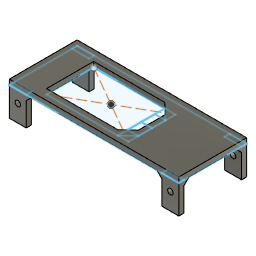
Power Rear Panel (Autodesk Fusion 360 design; units mm, degrees)
Autodesk Fusion 360 part; units mm, degrees
sketch "Sketch1" plane through (0, 0, 0) normal (0, 0, 1) x (1, 0, 0)
  line L0 (17.85, 0) -> (24.15, 0)
  line L1 (24.15, -8) -> (17.85, -13.9)
  line L2 (17.85, 8) -> (17.85, 0)
  line L3 (17.85, -13.9) -> (17.85, 13.9)
  line L4 (17.85, -8) -> (17.85, 0)
  line L5 (17.85, 0) -> (24.15, 0)
  line L6 (17.85, 13.9) -> (-24.15, 13.9)
  line L7 (24.15, 0) -> (24.15, -8)
  line L8 (-24.15, 13.9) -> (24.15, -13.9) construction
  line L9 (24.15, 8) -> (23.8007, 8)
  line L10 (24.15, -8) -> (17.85, -8)
  line L11 (24.15, 8) -> (17.85, 8)
  line L12 (24.15, 0) -> (24.15, 8)
  line L13 (17.85, 13.9) -> (24.15, 8)
  line L14 (-24.15, 13.9) -> (24.15, 13.9)
  line L15 (24.15, 13.9) -> (24.15, -13.9)
  line L16 (24.15, -13.9) -> (-24.15, -13.9)
  line L17 (-24.15, -13.9) -> (-24.15, 13.9)
  line L18 (24.15, 13.9) -> (-24.15, -13.9) construction
  line L19 (60, -20) -> (-40, -20)
  line L20 (-40, -20) -> (-40, 20)
  line L21 (-40, 20) -> (60, 20)
  line L22 (60, 20) -> (60, -20)
  line L23 (60, 20) -> (50, 20)
  line L24 (50, 20) -> (50, 17)
  line L25 (50, 17) -> (60, 17)
  line L26 (60, 17) -> (60, 20)
  line L27 (60, -20) -> (50, -20)
  line L28 (50, -20) -> (50, -17)
  line L29 (50, -17) -> (60, -17)
  line L30 (60, -17) -> (60, -20)
  line L31 (-40, -20) -> (-30, -20)
  line L32 (-30, -20) -> (-30, -17)
  line L33 (-30, -17) -> (-40, -17)
  line L34 (-40, -17) -> (-40, -20)
  line L35 (-40, 20) -> (-30, 20)
  line L36 (-30, 20) -> (-30, 17)
  line L37 (-30, 17) -> (-40, 17)
  line L38 (-40, 17) -> (-40, 20)
  dimension "d1" = 48.3
  dimension "d2" = 27.8
  dimension "d3" = 42
  dimension "d4" = 8
  dimension "d5" = 8
  dimension "d6" = 100
  dimension "d7" = 40
  dimension "d8" = 3
  dimension "d9" = 10
  dimension "d10" = 10
  dimension "d11" = 3
  dimension "d12" = 3
  dimension "d13" = 10
  dimension "d14" = 10
  dimension "d15" = 3
  dimension "d25" = 6.1
  dimension "d26" = 15.85
  constraint perpendicular L14 L15
  constraint parallel L14 L16
  constraint parallel L15 L17
  constraint horizontal L14
  constraint coincident origin L8
  constraint coincident origin L18
  constraint vertical L3
  constraint horizontal L6
  constraint horizontal L5
  constraint vertical L7
  constraint horizontal L10
  constraint vertical L4
  constraint midpoint L0.start L3
  constraint horizontal L0
  constraint vertical L12
  constraint horizontal L11
  constraint vertical L2
  constraint coincident L9.end L11
  constraint parallel L9 L11
  constraint perpendicular L19 L20
  constraint parallel L19 L21
  constraint parallel L20 L22
  constraint horizontal L19
  constraint horizontal L23
  constraint vertical L24
  constraint horizontal L25
  constraint vertical L26
  constraint horizontal L27
  constraint vertical L28
  constraint horizontal L29
  constraint vertical L30
  constraint horizontal L31
  constraint vertical L32
  constraint horizontal L33
  constraint vertical L34
  constraint horizontal L35
  constraint vertical L36
  constraint horizontal L37
  constraint vertical L38
  measures "d1" distance of L16.end L8.end
  measures "d2" distance of L14.end L8.end
  measures "d3" distance of L16.end L1.end
  measures "d4" distance of L4.start L0.start
  measures "d5" distance of L2.start L0.start
  measures "d6" distance of L20.end L21.end
  measures "d7" distance of L19.end L20.end
  measures "d8" distance of L21.end L25.end
  measures "d9" distance of L21.end L23.end
  measures "d10" distance of L19.start L27.end
  measures "d11" distance of L19.start L29.end
  measures "d12" distance of L19.end L33.end
  measures "d13" distance of L19.end L31.end
  measures "d14" distance of L20.end L35.end
  measures "d15" distance of L20.end L37.end
  measures "d25" distance of L14 L21
  measures "d26" distance of L17 L20
extrude "Extrude1" add sketch "Sketch1" along normal blind 3 contours L1 L15 L16 | L13 L14 L15 | L19 L22 L27 L28 L29 L30 | L19 L20 L21 L22 L24 L25 L28 L29 L32 L33 L36 L37 | L19 L20 L31 L32 L33 L34 | L21 L22 L23 L24 L25 L26 | L20 L21 L35 L36 L37 L38
extrude "Extrude2" add sketch "Sketch1" against normal blind 17 contours L19 L22 L27 L28 L29 L30 | L19 L20 L31 L32 L33 L34 | L21 L22 L23 L24 L25 L26 | L20 L21 L35 L36 L37 L38
sketch "Sketch2" plane through (0, 20, 0) normal (0, 1, 0) x (-1, 0, 0)
  line L0 (-50, 0) -> (30, 0)
  line L1 (30, 0) -> (30, -17)
  line L2 (30, -17) -> (40, -17)
  line L3 (40, -17) -> (40, 3)
  line L4 (40, 3) -> (-60, 3)
  line L5 (-60, 3) -> (-60, -17)
  line L6 (-60, -17) -> (-50, -17)
  line L7 (-50, -17) -> (-50, 0)
  circle A0 centre (35, -7) radius 1.625
  circle A1 centre (-55, -7) radius 1.625
  dimension "d20" = 3.25
  dimension "d21" = 3.25
  dimension "d27" = 5
  measures "d20" diameter of A0
  measures "d21" diameter of A1
  measures "d27" distance of L5 A1.centre
extrude "Extrude3" cut sketch "Sketch2" against normal up to surface (40 mm away) contours A0 | A1
chamfer "Chamfer1" distance 3 angle 45 8 edges at (-35, -17, 0) (-35, 17, 0) (55, -17, 0) (55, 17, 0) (50, 18.5, 0) (50, -18.5, 0) (-30, -18.5, 0) (-30, 18.5, 0)
